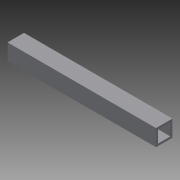
# Autodesk Inventor part: Part2
Saved by Autodesk Inventor 2015 (Build 190159000, 159)
## iProperties
Created: 2015-07-04
Part Number: Part2
Material: Generic
Document SubType Name: Modeling
Designer: tsayman
Density: 1 g/cm^3
Appearance: Default
Author: tsayman
Autodesk Inventor part; units mm, degrees
ref_plane "YZ Plane" through (0, 0, 0) normal (1, 0, 0) x (0, 1, 0)
ref_plane "XZ Plane" through (0, 0, 0) normal (0, 1, 0) x (-1, 0, 0)
ref_plane "XY Plane" through (0, 0, 0) normal (0, 0, 1) x (1, 0, 0)
sketch "Sketch1" plane through (0, 0, 0) normal (0, 0, 1) x (1, 0, 0)
  line L0 (-112.3194, 91.5028) -> (-340.9194, 91.5028)
  line L1 (-340.9194, 91.5028) -> (-340.9194, 66.1028)
  line L2 (-340.9194, 66.1028) -> (-112.3194, 66.1028)
  line L3 (-112.3194, 66.1028) -> (-112.3194, 91.5028)
  point P0 (0, 0)
  dimension "d0" = 228.6
  dimension "d1" = 25.4
  constraints: 8 end point, 2 parallel, 1 horizontal, 1 perpendicular
  measures "d0" distance of L1.end L2.end
  measures "d1" distance of L0.end L1.end
extrude "Extrusion1" add sketch "Sketch1" along normal blind 25.4
shell "Shell1" thickness 3.175 removed faces 2 at (-340.9194, 83.0362, 8.4667) at (-112.3194, 74.5695, 8.4667)
body "Solid1"
